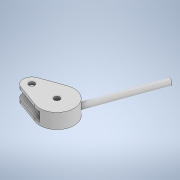
# Autodesk Inventor part: tumbler_holder
Saved by Autodesk Inventor 2021 (Build 250183000, 183)
## iProperties
Created: 2024-11-04
Part Number: tumbler_holder
Material: Generic
Document SubType Name: Modeling
Designer: sriva
Density: 1 g/cm^3
Appearance: Default
Author: sriva
Autodesk Inventor part; units mm, degrees
sketch "Sketch1" plane through (0, 0, 0) normal (0, 1, 0) x (-1, 0, 0)
  circle A0 centre (-12.4151, -0.0018) radius 20
  line L0 (-12.4151, -0.0018) -> (-56.4151, -0.0018)
  circle A1 centre (-56.4151, -0.0018) radius 24
  circle A2 centre (-12.4151, -0.0018) radius 15
  circle A3 centre (-56.4151, -0.0018) radius 27.5
  circle A4 centre (-56.4151, -0.0018) radius 30
  line L1 (-56.4151, 29.9982) -> (-56.4151, -30.0018)
  line L2 (-44.4256, 27.4982) -> (-7.3229, 14.1074)
  line L3 (-44.4256, -27.5018) -> (-7.3229, -14.111)
  point P0 (2.5568, 7.0507)
  point P1 (-7.3015, 14.0996)
  point P2 (-40.9628, 25.7125)
  point P3 (-26.7447, -4.4362)
  point P4 (-26.7447, 4.4326)
  point P5 (-26.7447, -4.4362)
  point P6 (-26.7447, 4.4326)
  dimension "d2" = 40
  dimension "d3" = 44
  dimension "d4" = 30
  dimension "d5" = 55
  dimension "d8" = 60
  constraints: 8 end point, 6 point on circle, 5 centre point, 4 coincident, 2 symmetric about line, 1 horizontal
  measures "d2" diameter of A0
  measures "d3" distance of L0.start L0.end
  measures "d4" diameter of A2
  measures "d5" diameter of A3
  measures "d8" diameter of A4
extrude "Extrusion1" add sketch "Sketch1" along normal blind 5 contours L2 A2 A4 A0 | A0 A4 L2 | L3 A4 A0 | A0 A4 A2 L3 | A4 A2 L0 A3 A0 | A0 A3 L1 A4 | A2 A4 | A4 L1 A3 A0 | A0 A3 L0 A2 A4 | A3 L0 A0 | A0 A1 L1 A3 | A4 L0 A2 | L1 A3 A4 | A3 L1 A1 A0 | A0 L0 A3 | A2 L0 A4 | A1 L1 L0 | L0 L1 A1 | L1 A1 A3 | L1 A1
ref_plane "Work Plane1" through (0, 5, 0) normal (0, -1, 0) x (1, 0, 0)
ref_plane "Work Plane2" through (0, 21, 0) normal (0, -1, 0) x (1, 0, 0)
sketch "Sketch4" plane through (0, 21, 0) normal (0, -1, 0) x (1, 0, 0)
  arc A0 (7.3229, 14.1074) -> (7.3229, -14.111) centre (12.4151, -0.0018) ccw projected
  circle A1 centre (12.4151, -0.0018) radius 7.5
  circle A2 centre (56.4151, -0.0018) radius 17.5
  arc A3 (7.3229, 14.1074) -> (7.3229, -14.111) centre (12.4151, -0.0018) ccw projected
  line L0 (7.3015, 14.0996) -> (39.6751, 27.8553) projected
  line L1 (7.3015, 14.0996) -> (39.6751, 27.8553)
  line L2 (39.6751, -27.8589) -> (7.3015, -14.1032) projected
  line L3 (7.3015, -14.1032) -> (39.6751, -27.8589)
  line L4 (7.3229, 14.1074) -> (44.4256, 27.4982) projected
  line L5 (44.4256, -27.5018) -> (7.3229, -14.111) projected
  arc A4 (44.4256, -27.5018) -> (44.4256, 27.4982) centre (56.4151, -0.0018) ccw projected
  point P0 (0, 0)
  constraints: 4 end point, 2 centre point, 2 collinear, 1 coincident
extrude "Extrusion3" add sketch "Sketch4" against normal blind 5 contours L4 A4 L5 A0 | A1 | A2
sketch "Sketch5" plane through (0, 26, 0) normal (0, 1, 0) x (1, 0, 0)
  line L0 (0, 0) -> (-2.5, 0)
  arc A0 (44.4256, -27.4982) -> (44.4256, 27.5018) centre (56.4151, 0.0018) ccw projected
  line L1 (56.4151, 0.0018) -> (53.9151, 0.0018)
  line L2 (44.4256, 27.5018) -> (7.3229, 14.111) projected
  arc A1 (7.3229, 14.111) -> (7.3229, -14.1074) centre (12.4151, 0.0018) ccw projected
  line L3 (7.3229, -14.1074) -> (44.4256, -27.4982) projected
  circle A2 centre (12.4151, 0.0018) radius 5
  circle A3 centre (56.4151, 0.0018) radius 5
  point P0 (12.9861, -15)
  point P1 (12.9861, 15)
  dimension "d29" = 10
  dimension "d30" = 10
  constraints: 4 end point, 2 centre point, 2 coincident, 2 horizontal
  measures "d29" diameter of A2
  measures "d30" diameter of A3
extrude "Extrusion4" cut sketch "Sketch5" against normal through all contours A2 | A3
ref_plane "Work Plane4" through (0, 5, 0) normal (0, -1, 0) x (1, 0, 0)
sketch "Sketch8" plane through (0, 5, 0) normal (0, -1, 0) x (1, 0, 0)
  line L0 (44.4256, -27.5018) -> (7.3229, -14.111) projected
  arc A0 (7.3229, 14.1074) -> (7.3229, -14.111) centre (12.4151, -0.0018) ccw projected
  line L1 (7.3229, 14.1074) -> (44.4256, 27.4982) projected
  arc A1 (44.4256, -27.5018) -> (44.4256, 27.4982) centre (56.4151, -0.0018) ccw projected
  circle A2 centre (56.4151, -0.0018) radius 5 projected
  circle A3 centre (56.4151, -0.0018) radius 27.5
  arc A4 (44.4256, -27.5018) -> (44.4256, 27.4982) centre (56.4151, -0.0018) ccw projected
  line L2 (56.4151, -30.0018) -> (56.4151, 29.9982)
  point P0 (0, 0)
  point P1 (56.4151, 27.4982)
  point P2 (56.4151, -27.5018)
  dimension "d32" = 55
  constraints: 2 end point, 2 point on circle, 1 centre point, 1 coincident, 1 vertical
  measures "d32" diameter of A3
extrude "Extrusion7" add sketch "Sketch8" against normal up to surface (16 mm away) contours L2 A3 A1
ref_plane "Work Plane5" through (66.5995, 21, -28.2202) normal (-0.3394792, 0, 0.9406136) x (0, -1, 0)
sketch "Sketch9" plane through (66.5995, 21, -28.2202) normal (-0.3394792, 0, 0.9406136) x (0, -1, 0)
  line L0 (16, 10.1844) -> (0, 10.1844) projected
  circle A0 centre (8, 10.1844) radius 5
  point P0 (21, -53.0642)
  dimension "d35" = 10
  constraints: 1 centre point, 1 midpoint
  measures "d35" diameter of A0
extrude "Extrusion8" add sketch "Sketch9" along normal up to surface round surface about axis through (56.4151, 21, -0.0018) along (0, 1, 0) radius 30 far side no
sketch "Sketch10" plane through (76.1791, 13, -24.7628) normal (0.3394792, 0, -0.9406136) x (-0.9406136, 0, -0.3394792)
  line L0 (0, -8) -> (0, 8) projected
  circle A0 centre (0, 0) radius 5
  point P0 (63.2486, -13)
  constraints: 1 centre point, 1 midpoint
extrude "Extrusion9" add sketch "Sketch10" along normal blind 120
body "Solid1"
